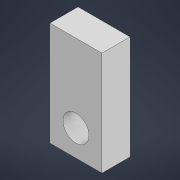
# Autodesk Inventor part: Circle_TestFit_V1
Saved by Autodesk Inventor 2022 (Build 260153000, 153)
## iProperties
Created: 2023-05-10
Part Number: Circle_TestFit_V1
Material: Generic
Document SubType Name: Modeling
Designer: Karl Spiteri
Density: 1 g/cm^3
Appearance: Default
Author: Karl Spiteri
Autodesk Inventor part; units mm, degrees
ref_plane "YZ Plane" through (0, 0, 0) normal (1, 0, 0) x (0, 1, 0)
ref_plane "XZ Plane" through (0, 0, 0) normal (0, 1, 0) x (-1, 0, 0)
ref_plane "XY Plane" through (0, 0, 0) normal (0, 0, 1) x (1, 0, 0)
sketch "Sketch4" plane through (0, 0, 0) normal (0, 0, 1) x (1, 0, 0)
  line L0 (0, 0) -> (-10, 0)
  line L1 (-10, 0) -> (-10, 20)
  line L2 (-10, 20) -> (0, 20)
  line L3 (0, 20) -> (0, 0)
  dimension "d22" = 10
  dimension "d23" = 20
  constraints: 8 end point, 2 parallel, 1 horizontal, 1 perpendicular
  measures "d22" distance of L1.end L2.end
  measures "d23" distance of L0.end L1.end
extrude "Extrusion3" add sketch "Sketch4" along normal blind 5.4
sketch "Sketch5" plane through (0, 0, 5.4) normal (0, 0, 1) x (1, 0, 0)
  point P0 (0, 0)
  point P1 (-5, 5)
hole "Hole3" at (-5, 5, 5.4) direction (0, 0, -1) diameter 5 depth 6
body "Solid3"
